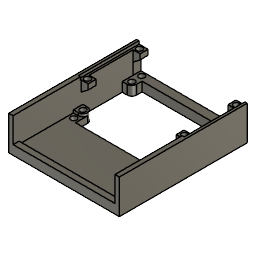
main (Autodesk Fusion 360 design; units mm, degrees)
Autodesk Fusion 360 part; units mm, degrees
note: some values were not read from the file. Set by a fixed rule: which sketch regions a step uses.
sketch "Szkic1" plane through (0, 0, 0) normal (0, 0, 1) x (1, 0, 0)
  line L0 (7.004, 84.481) -> (7.004, 88.113)
  arc A0 (3.502, 80.979) -> (7.004, 84.481) centre (3.502, 84.481) ccw
  line L1 (0, 80.979) -> (3.502, 80.979)
  line L2 (0, 0) -> (0, 88.113)
  line L3 (-0.2, 0) -> (-0.2, 88.113)
  line L4 (-3.5, 0) -> (-3.5, 88.113)
  line L5 (-3.5, 89.113) -> (-3.5, 95.113)
  line L6 (0, 95.113) -> (-3.5, 95.113)
  line L7 (-3.5, 89.113) -> (-3.5, 88.113)
  line L8 (0, 88.113) -> (76.073, 88.113)
  line L9 (-0.2, 88.113) -> (-0.2, 89.113)
  line L10 (0, 95.113) -> (76.073, 95.113)
  line L11 (76.273, 89.113) -> (76.273, 95.113)
  line L12 (76.073, 88.113) -> (76.073, 0)
  line L13 (76.273, 88.113) -> (76.273, 89.113)
  line L14 (76.273, 0) -> (76.273, 88.113)
  circle A1 centre (72.571, 84.481) radius 2.25
  arc A2 (69.069, 84.481) -> (72.571, 80.979) centre (72.571, 84.481) ccw
  line L15 (69.069, 84.481) -> (69.069, 88.113)
  line L16 (76.073, 80.979) -> (72.571, 80.979)
  circle A3 centre (3.502, 84.481) radius 2.25
  line L17 (0, -1) -> (-3.5, -1)
  line L18 (-3.5, -1) -> (-3.5, 0)
  line L19 (-0.2, 0) -> (-0.2, -1)
  line L20 (76.073, 0) -> (0, 0)
  line L21 (76.073, -1) -> (0, -1)
  arc A4 (3.502, 44.277) -> (3.502, 51.281) centre (3.502, 47.779) ccw
  line L22 (3.502, 51.281) -> (0, 51.281)
  line L23 (3.502, 44.277) -> (0, 44.277)
  circle A5 centre (3.502, 47.779) radius 2.25
  line L24 (72.571, 51.281) -> (76.073, 51.281)
  line L25 (72.571, 44.277) -> (76.073, 44.277)
  arc A6 (72.571, 51.281) -> (72.571, 44.277) centre (72.571, 47.779) ccw
  circle A7 centre (72.571, 47.779) radius 2.25
  line L26 (79.573, 88.113) -> (79.573, 0)
  line L27 (76.073, 95.113) -> (79.573, 95.113)
  line L28 (79.573, 95.113) -> (79.573, 89.113)
  line L29 (79.573, 89.113) -> (79.573, 88.113)
  line L30 (79.573, -1) -> (79.573, 0)
  line L31 (76.273, 0) -> (76.273, -1)
  line L32 (76.073, -1) -> (79.573, -1)
  line L33 (-0.2, 89.113) -> (-0.2, 95.113)
  line L34 (0, 88.113) -> (-0.2, 88.113)
  line L35 (76.073, 88.113) -> (76.273, 88.113)
  line L36 (76.073, 0) -> (76.273, 0)
  line L37 (0, 0) -> (-0.2, 0)
  line L38 (73.073, 0) -> (73.073, 3.5)
  line L39 (73.073, 3.5) -> (76.073, 3.5)
  line L40 (38.0365, 101.5763) -> (38.0365, -20) construction
  line L41 (3, 0) -> (3, 3.5)
  line L42 (3, 3.5) -> (0, 3.5)
  line L43 (69.069, 88.113) -> (69.069, 95.113)
  line L44 (7.004, 88.113) -> (7.004, 95.113)
  line L45 (82, 66.13) -> (-9, 66.13) construction
  circle A8 centre (3.502, 91.9192) radius 2.25
  circle A9 centre (3.502, 40.9192) radius 2.25
  circle A10 centre (72.571, 91.9192) radius 2.25
  circle A11 centre (72.571, 40.9192) radius 2.25
  line L46 (0, 3.5) -> (-0.2, 3.5)
  line L47 (76.073, 3.5) -> (76.273, 3.5)
  line L48 (0, 80.979) -> (-0.2, 80.979)
  line L49 (76.073, 80.979) -> (76.273, 80.979)
  line L50 (0, 44.277) -> (-0.2, 44.277)
  line L51 (0, 51.281) -> (-0.2, 51.281)
  line L52 (76.073, 51.281) -> (76.273, 51.281)
  line L53 (76.073, 44.277) -> (76.273, 44.277)
  line L54 (3, 3.5) -> (73.073, 3.5)
  dimension "d3" = 3
  dimension "d4" = 4.5
  dimension "d5" = 4.5
  dimension "d48" = 51
  constraint coincident L2.end L8.start
  constraint coincident L3.end L9.start
  constraint coincident L8.end L12.start
  constraint coincident L13.start L14.end
  constraint coincident L12.end L20.start
  constraint coincident L14.start L31.start
  constraint coincident L2.start L20.end
  constraint coincident L3.start L19.start
  constraint coincident L20 L38.start
  constraint perpendicular L20 L38
  constraint coincident L12 L39.end
  constraint perpendicular L12 L39
  constraint perpendicular L20 L40
  constraint symmetric L38.start L40 L41.start
  constraint symmetric L38.end L40 L41.end
  constraint symmetric L39.end L40 L42.end
  constraint coincident L15.end L43.start
  constraint coincident L10 L43.end
  constraint perpendicular L10 L43
  constraint coincident L0.end L44.start
  constraint coincident L10 L44.end
  constraint perpendicular L10 L44
  constraint perpendicular L4 L45
  constraint symmetric A3 A5 L45
  constraint symmetric L40 A8 A10
  constraint symmetric L40 A9 A11
  constraint coincident L3 L46.end
  constraint perpendicular L3 L46
  constraint coincident L14 L47.end
  constraint perpendicular L14 L47
  constraint coincident L1.start L48.start
  constraint coincident L3 L48.end
  constraint perpendicular L3 L48
  constraint coincident L16.start L49.start
  constraint perpendicular L14 L49
  constraint coincident L23.end L50.start
  constraint coincident L3 L50.end
  constraint perpendicular L3 L50
  constraint coincident L22.end L51.start
  constraint coincident L3 L51.end
  constraint perpendicular L3 L51
  constraint coincident L24.end L52.start
  constraint coincident L14 L52.end
  constraint perpendicular L14 L52
  constraint coincident L25.end L53.start
  constraint coincident L14 L53.end
  constraint perpendicular L14 L53
  measures "d3" distance of L38.end L39.end
  measures "d4" diameter of A8
  measures "d5" diameter of A9
  measures "d48" distance of A10.centre A11.centre
extrude "Wyciągnięcie proste2" add sketch "Szkic1" along normal blind 5
extrude "Wyciągnięcie proste3" add sketch "Szkic1" along normal blind 7 contours L0 A0 L1 L2 L8 | L8 L10 L43 L44 | L6 L8 L9 L10 L33 L34 L44 | L2 L3 L34 L48 | L8 L10 L11 L13 L27 L35 L43 | L8 L12 A2 L15 L16 | L3 L4 L5 L6 L7 L9 L17 L18 L19 L33 | L12 L14 L35 L49 | L2 A4 L22 L23 | L2 L3 L50 L51 | L11 L13 L14 L26 L27 L28 L29 L30 L31 L32 | L12 L14 L52 L53 | L12 L24 L25 A6 | L2 L20 L41 L42 | L2 L3 L37 L46 | L17 L19 L20 L21 L31 L32 L36 L37 | L12 L14 L36 L47 | L12 L20 L38 L39
extrude "Wyciągnięcie proste4" add sketch "Szkic1" along normal blind 25.8 contours L3 L4 L5 L6 L7 L9 L17 L18 L19 L33 | L11 L13 L14 L26 L27 L28 L29 L30 L31 L32
sketch "Szkic2" plane through (0, 95.113, 0) normal (0, 1, 0) x (-1, 0, 0)
  line L0 (-79.573, 0) -> (0, 0)
  line L1 (0, 0) -> (0, 7)
  line L2 (0, 7) -> (-76.273, 7)
  line L3 (-76.273, 7) -> (-76.273, 25.8)
  line L4 (-76.273, 25.8) -> (-79.573, 25.8)
  line L5 (-79.573, 25.8) -> (-79.573, 0)
sketch "Szkic3" plane through (0, 95.113, 0) normal (0, 1, 0) x (-1, 0, 0)
  line L0 (-79.573, 0) -> (0, 0)
  line L1 (0, 0) -> (0, 7)
  line L2 (0, 7) -> (-76.273, 7)
  line L3 (-76.273, 7) -> (-76.273, 25.8)
  line L4 (-76.273, 25.8) -> (-79.573, 25.8)
  line L5 (-79.573, 25.8) -> (-79.573, 0)
  line L6 (-38.0365, 31.6358) -> (-38.0365, -19.2) construction
  line L7 (-76.273, 23.6) -> (-69.069, 23.6)
  line L8 (-69.069, 23.6) -> (-69.069, 20.804)
  line L9 (-76.273, 13.6) -> (-76.273, 23.6)
  line L10 (-76.273, 25.8) -> (-79.573, 25.8)
  line L11 (-76.273, 13.6) -> (-69.069, 20.804)
  line L12 (-76.273, 13.6) -> (-66.085, 13.6) construction
  line L13 (0.2, 23.6) -> (-7.004, 23.6)
  line L14 (0.2, 13.6) -> (-7.004, 20.804)
  line L15 (-7.004, 23.6) -> (-7.004, 20.804)
  line L16 (0.2, 13.6) -> (0.2, 23.6)
  dimension "d12" = 10
  dimension "d13" = 2.2
  dimension "d14" = 45
  constraint perpendicular L0 L6
  constraint horizontal L7
  constraint vertical L8
  constraint vertical L9
  constraint coincident L3 L7.start
  constraint horizontal L12
  constraint symmetric L6 L7.start L13.start
  constraint symmetric L6 L7.end L13.end
  constraint symmetric L6 L9.start L14.start
  constraint symmetric L6 L8.end L14.end
  measures "d12" distance of L7.start L9.start
  measures "d13" distance of L7 L10
  measures "d14" angle of L11 L12
extrude "Wyciągnięcie proste5" add sketch "Szkic3" against normal blind 7 contours L3 L7 L8 L9 L11 | L13 L14 L15 L16
sketch "Szkic4" plane through (0, 0, 23.6) normal (0, 0, 1) x (-1, 0, 0)
  line L0 (-76.273, -95.113) -> (-69.069, -95.113)
  line L1 (-69.069, -95.113) -> (-69.069, -88.113)
  line L2 (-69.069, -88.113) -> (-76.273, -88.113)
  line L3 (-76.273, -88.113) -> (-76.273, -95.113)
  circle A0 centre (-74.5365, -92.113) radius 2.25
  line L4 (-76.273, -95.113) -> (-77.7365, -95.113)
  line L5 (-77.7365, -95.113) -> (-77.7365, -50.113)
  line L6 (-77.7365, -50.113) -> (-76.273, -50.113)
  line L7 (-76.273, -56.113) -> (-76.273, -50.113)
  circle A1 centre (-74.5365, -53.113) radius 2.25
  line L8 (-78.0365, -95.113) -> (-71.0365, -95.113)
  line L9 (-71.0365, -95.113) -> (-71.0365, -89.113)
  line L10 (-71.0365, -89.113) -> (-78.0365, -89.113)
  line L11 (-78.0365, -89.113) -> (-78.0365, -95.113)
  line L12 (-78.0365, -95.113) -> (-71.0365, -89.113) construction
  line L13 (-71.0365, -95.113) -> (-78.0365, -89.113) construction
  line L14 (-78.0365, -50.113) -> (-71.0365, -50.113)
  line L15 (-71.0365, -50.113) -> (-71.0365, -56.113)
  line L16 (-71.0365, -56.113) -> (-78.0365, -56.113)
  line L17 (-78.0365, -56.113) -> (-78.0365, -50.113)
  line L18 (-78.0365, -50.113) -> (-71.0365, -56.113) construction
  line L19 (-71.0365, -50.113) -> (-78.0365, -56.113) construction
  line L20 (-76.273, -95.113) -> (0, -95.113) construction
  line L21 (-38.0365, -105.87) -> (-38.0365, 20) construction
  line L22 (1.9635, -95.113) -> (-5.0365, -95.113)
  line L23 (-5.0365, -95.113) -> (-5.0365, -89.113)
  line L24 (-5.0365, -89.113) -> (1.9635, -89.113)
  circle A2 centre (-1.5365, -92.113) radius 2.25
  line L25 (1.6635, -95.113) -> (1.6635, -50.113)
  line L26 (-5.0365, -56.113) -> (1.9635, -56.113)
  line L27 (-5.0365, -50.113) -> (-5.0365, -56.113)
  line L28 (1.9635, -50.113) -> (-5.0365, -50.113)
  circle A3 centre (-1.5365, -53.113) radius 2.25
  line L29 (-76.273, -89.113) -> (-76.273, -56.113)
  line L30 (-76.273, -56.113) -> (-76.273, -89.113)
  line L31 (-76.273, -89.113) -> (-76.273, -95.113)
  line L32 (-77.7365, -95.113) -> (-77.7365, -50.113)
  line L33 (-76.273, -50.113) -> (-76.273, -56.113)
  line L34 (-76.273, -50.113) -> (-77.7365, -50.113)
  line L35 (-76.273, -95.113) -> (-76.273, -93.5438)
  line L36 (-76.273, -89.113) -> (-76.273, -90.6822)
  line L37 (-76.273, -95.113) -> (-71.0365, -95.113)
  line L38 (-76.273, -89.113) -> (-71.0365, -89.113)
  line L39 (-76.273, -56.113) -> (-71.0365, -56.113)
  line L40 (-71.0365, -56.113) -> (-76.273, -56.113)
  line L41 (-71.0365, -50.113) -> (-76.273, -50.113)
  line L42 (-76.273, -50.113) -> (-76.273, -51.6822)
  line L43 (-76.273, -56.113) -> (-76.273, -54.5438)
  line L44 (-5.0365, -56.113) -> (0.2, -56.113)
  line L45 (0.2, -56.113) -> (0.2, -89.113)
  line L46 (0.2, -56.113) -> (0.2, -54.5438)
  line L47 (-5.0365, -50.113) -> (-5.0365, -56.113)
  line L48 (-5.0365, -50.113) -> (0.2, -50.113)
  circle A4 centre (-1.5365, -53.113) radius 2.25
  line L49 (0.2, -50.113) -> (0.2, -51.6822)
  line L50 (1.6635, -50.113) -> (0.2, -50.113)
  line L51 (1.6635, -95.113) -> (1.6635, -50.113)
  line L52 (0.2, -95.113) -> (1.6635, -95.113)
  line L53 (0.2, -95.113) -> (-5.0365, -95.113)
  circle A5 centre (-1.5365, -92.113) radius 2.25
  line L54 (0.2, -95.113) -> (0.2, -93.5438)
  line L55 (0.2, -89.113) -> (0.2, -90.6822)
  line L56 (-5.0365, -95.113) -> (-5.0365, -89.113)
  line L57 (0.2, -89.113) -> (-5.0365, -89.113)
  line L58 (-71.0365, -50.113) -> (-77.7365, -50.113)
  line L59 (-77.7365, -50.113) -> (-77.7365, -49.613)
  line L60 (-77.7365, -49.613) -> (-71.0365, -49.613)
  line L61 (-71.0365, -49.613) -> (-71.0365, -50.113)
  line L62 (-5.0365, -49.613) -> (-5.0365, -50.113)
  line L63 (1.6635, -49.613) -> (-5.0365, -49.613)
  line L64 (1.6635, -50.113) -> (1.6635, -49.613)
  point P0 (-74.5365, -92.113)
  point P1 (-74.5365, -53.113)
  dimension "d17" = 4.5
  dimension "d19" = 3
  dimension "d20" = 45
  dimension "d21" = 3.2
  dimension "d23" = 4.5
  dimension "d24" = 39
  dimension "d29" = 7
  dimension "d30" = 7
  dimension "d31" = 6
  dimension "d32" = 36.5
  dimension "d37" = 0.5
  constraint horizontal L4
  constraint vertical L5
  constraint horizontal L6
  constraint coincident L0.start L3.end
  constraint vertical L7
  constraint horizontal L8
  constraint perpendicular L8 L9
  constraint parallel L8 L10
  constraint parallel L9 L11
  constraint coincident L12 P0
  constraint coincident L13 P0
  constraint coincident P0 A0.centre
  constraint horizontal L14
  constraint perpendicular L14 L15
  constraint parallel L14 L16
  constraint parallel L15 L17
  constraint coincident L18 P1
  constraint coincident L19 P1
  constraint coincident P1 A1.centre
  constraint perpendicular L20 L21
  constraint symmetric A0 L21 A2
  constraint symmetric L4.end L21 L25.start
  constraint symmetric L5.end L21 L25.end
  constraint symmetric A1 L21 A3
  constraint symmetric L8.start L21 L22.start
  constraint symmetric L8.end L21 L22.end
  constraint symmetric L9.end L21 L23.end
  constraint symmetric L10.end L21 L24.end
  constraint symmetric L14.start L21 L28.start
  constraint symmetric L14.end L21 L27.start
  constraint symmetric L15.end L21 L26.start
  constraint symmetric L16.end L21 L26.end
  constraint coincident L10 L29.start
  constraint coincident L3 L29.start
  constraint perpendicular L16 L29
  constraint coincident A0 L35.end
  constraint coincident L31 L35.end
  constraint coincident A0 L36.end
  constraint coincident L31 L36.end
  constraint perpendicular L9 L37
  constraint perpendicular L15 L39
  constraint perpendicular L7 L41
  constraint coincident A1 L42.end
  constraint coincident L7 L42.end
  constraint coincident A1 L43.end
  constraint coincident L7 L43.end
  constraint symmetric A0 L21 A5
  constraint symmetric L0.start L21 L52.start
  constraint symmetric L6.end L21 L48.end
  constraint symmetric L7.start L21 L44.end
  constraint symmetric A1 L21 A4
  constraint symmetric L21 L29.start L45.end
  constraint symmetric L21 L35.end L54.end
  constraint symmetric L21 L36.end L55.end
  constraint symmetric L21 L0.start L52.start
  constraint symmetric L21 L42.end L49.end
  constraint symmetric L21 L43.end L46.end
  constraint horizontal L58
  constraint vertical L59
  constraint horizontal L60
  constraint vertical L61
  constraint symmetric L21 L5.end L25.end
  constraint symmetric L21 L59.end L63.start
  constraint symmetric L21 L60.end L62.start
  measures "d17" diameter of A0
  measures "d19" distance of L0 P0
  measures "d20" distance of L0.start L6.end
  measures "d21" distance of P0 L5
  measures "d23" diameter of A1
  measures "d24" distance of P0 P1
  measures "d29" distance of L9.end L10.end
  measures "d30" distance of L15.end L16.end
  measures "d31" distance of L14.end L15.end
  measures "d32" distance of P0 L21
  measures "d37" distance of L14.end L60.end
extrude "Wyciągnięcie proste6" cut sketch "Szkic4" 1 faces at (4.6027, 90.7797, 23.6) against normal blind 10 contours L0 L3 A0 L8 L9 L10 L31 L35 L36 L37 L38 | L0 L1 L2 L3 L9 L10 L29 L30 L38 | L3 A0 L31 picked at (-73.0917, -91.9544)
extrude "Wyciągnięcie proste7" cut sketch "Szkic4" along normal blind 4 contours L3 A0 L4 L5 L8 L10 L31 L32 L35 L36 | L3 A0 L31 | L3 A0 L31 | L3 L5 L10 L16 L29 L30 L32 | L5 L6 L7 A1 L14 L16 L32 L33 L34 L42 L43 L58 | L6 L14 L34 L41 L58 L59 L60 L61 | L7 A1 L33 | L7 A1 L33 | L22 L24 A2 L25 L51 L52 A5 L54 L55 | L24 L25 L26 L45 L51 | A2 A5 | L25 L26 L28 A3 L46 A4 L49 L50 L51 | L28 L48 L50 L62 L63 L64 | A3 A4
extrude "Wyciągnięcie proste8" cut sketch "Szkic4" against normal blind 8 contours L3 A0 L31 | L3 A0 L31 | L7 A1 L33 | L7 A1 L33 | A2 A5 | A3 A4
extrude "Wyciągnięcie proste9" add sketch "Szkic4" against normal blind 8 contours L0 L3 A0 L8 L9 L10 L31 L35 L36 L37 L38 | L7 A1 L14 L15 L16 L33 L39 L40 L41 L42 L43 L58 | L22 L23 L24 A2 L53 A5 L54 L55 L56 L57 | L26 L27 L28 A3 L44 L46 L47 L48 A4 L49
sketch "Szkic5" plane through (0, 95.113, 0) normal (0, 1, 0) x (-1, 0, 0)
  line L0 (-77.7365, 23.6) -> (-77.7365, 25.8)
  line L1 (-77.7365, 25.8) -> (-79.573, 25.8)
  line L2 (-79.573, 25.8) -> (-79.573, 0)
  line L3 (-79.573, 0) -> (0, 0)
  line L4 (0, 0) -> (0, 7)
  line L5 (0, 7) -> (-76.273, 7)
  line L6 (-76.273, 7) -> (-76.273, 15.6)
  line L7 (-76.273, 15.6) -> (-71.0365, 15.6)
  line L8 (-71.0365, 15.6) -> (-71.0365, 23.6)
  line L9 (-71.0365, 23.6) -> (-77.7365, 23.6)
  line L10 (-76.273, 15.6) -> (-71.0365, 19.6)
  line L11 (-69.069, 5) -> (-7.004, 5) construction
  line L12 (-38.0365, 29.2995) -> (-38.0365, -9) construction
  line L13 (0.2, 15.6) -> (-5.0365, 19.6)
  line L14 (-5.0365, 23.6) -> (-5.0365, 15.6) construction
  line L15 (-5.0365, 19.6) -> (-5.0365, 15.6)
  line L16 (-5.0365, 15.6) -> (0.2, 15.6)
  point P0 (-5.0365, 15.6)
  constraint coincident L6.end L7.start
  constraint midpoint L8 L10.end
  constraint perpendicular L11 L12
  constraint symmetric L6.end L12 L13.start
  constraint symmetric L10.end L12 L13.end
  constraint coincident P0 L14.end
  constraint parallel L14 L15
extrude "Wyciągnięcie proste10" cut sketch "Szkic5" against normal blind 52 contours L7 L8 L10 | L13 L15 L16
sketch "Szkic6" plane through (0, 0, 0) normal (0, 0, -1) x (1, 0, 0)
  circle A0 centre (72.571, -47.779) radius 2.25
  circle A1 centre (3.502, -84.481) radius 2.25
  circle A2 centre (72.571, -91.9192) radius 2.25
  circle A3 centre (3.502, -91.9192) radius 2.25
  circle A4 centre (3.502, -47.779) radius 2.25
  circle A5 centre (72.571, -84.481) radius 2.25
  circle A6 centre (3.502, -40.9192) radius 2.25
  circle A7 centre (72.571, -40.9192) radius 2.25
  line L0 (79.573, 1) -> (-3.5, 1)
  line L1 (-3.5, 1) -> (-3.5, 0)
  line L2 (-3.5, 0) -> (-3.5, -88.113)
  line L3 (-3.5, -88.113) -> (-3.5, -89.113)
  line L4 (-3.5, -89.113) -> (-3.5, -95.113)
  line L5 (-3.5, -95.113) -> (0, -95.113)
  line L6 (0, -95.113) -> (79.573, -95.113)
  line L7 (79.573, -95.113) -> (79.573, 1)
  circle A8 centre (72.571, -91.9192) radius 3.502
  line L8 (69.069, -88.113) -> (69.069, -95.113)
  line L9 (38.0365, -94.1692) -> (72.571, -94.1692)
  arc A9 (72.571, -44.277) -> (72.571, -51.281) centre (72.571, -47.779) ccw
  line L10 (69.069, -47.779) -> (69.069, -40.9192)
  line L11 (38.0365, -38.6692) -> (72.571, -38.6692)
  line L12 (69.069, -40.9192) -> (69.069, -38.6692)
  line L13 (38.0365, -101.5763) -> (38.0365, 20) construction
  line L14 (38.0365, -94.1692) -> (3.502, -94.1692)
  line L15 (7.004, -47.779) -> (7.004, -40.9192)
  line L16 (7.004, -40.9192) -> (7.004, -38.6692)
  line L17 (38.0365, -38.6692) -> (3.502, -38.6692)
  line L18 (7.004, -94.1692) -> (69.069, -94.1692)
  line L19 (69.069, -94.1692) -> (69.069, -88.113)
  line L20 (7.004, -88.113) -> (7.004, -94.1692)
  line L21 (72.571, -51.281) -> (76.073, -51.281)
  line L22 (76.073, -51.281) -> (76.073, -80.979)
  arc A10 (72.571, -80.979) -> (69.069, -84.481) centre (72.571, -84.481) ccw
  line L23 (76.073, -80.979) -> (72.571, -80.979)
  line L24 (69.069, -88.113) -> (69.069, -84.481)
  arc A11 (72.571, -80.979) -> (69.069, -84.481) centre (72.571, -84.481) ccw
  arc A12 (71.864, -44.3491) -> (73.278, -44.3491) centre (72.571, -40.9192) ccw
  line L25 (69.069, -40.9192) -> (69.069, -38.6692)
  arc A13 (69.069, -47.779) -> (72.571, -51.281) centre (72.571, -47.779) ccw
  arc A14 (73.278, -44.3491) -> (71.864, -44.3491) centre (72.571, -47.779) ccw
  line L26 (38.0365, -101.5763) -> (38.0365, 20)
  line L27 (0, -51.281) -> (0, -80.979)
  line L28 (3.502, -51.281) -> (0, -51.281)
  arc A15 (3.502, -51.281) -> (7.004, -47.779) centre (3.502, -47.779) ccw
  line L29 (7.004, -47.779) -> (7.004, -40.9192)
  line L30 (7.004, -40.9192) -> (7.004, -38.6692)
  line L31 (0, -80.979) -> (3.502, -80.979)
  arc A16 (7.004, -84.481) -> (3.502, -80.979) centre (3.502, -84.481) ccw
  line L32 (7.004, -88.113) -> (7.004, -84.481)
  line L33 (7.004, -88.6692) -> (38.0365, -88.6692)
  line L34 (69.069, -88.6692) -> (38.0365, -88.6692)
  point P0 (38.0365, -101.5763)
  point P1 (76.073, -51.281)
  point P2 (76.073, -80.979)
  dimension "d50" = 50
  constraint concentric A2 A8
  constraint tangent A8 L8
  constraint coincident A2 L9.end
  constraint tangent A2 L9
  constraint concentric A7 A12
  constraint midpoint A9 L10.start
  constraint tangent L10 A12
  constraint vertical L10
  constraint coincident A7 L11.end
  constraint tangent A7 L11
  constraint coincident L11 L12.end
  constraint tangent L12 A12
  constraint coincident P0 L13.start
  constraint perpendicular L0 L13
  constraint coincident L9.start L13
  constraint perpendicular L9 L13
  constraint coincident L11.start L13
  constraint perpendicular L11 L13
  constraint symmetric L9.start L13 L14.start
  constraint symmetric L9.end L13 L14.end
  constraint symmetric L10.start L13 L15.start
  constraint symmetric L10.end L13 L15.end
  constraint symmetric L11.start L13 L17.start
  constraint symmetric L11.end L13 L17.end
  constraint symmetric L12.end L13 L16.end
  constraint horizontal L18
  constraint vertical L19
  constraint vertical L20
  constraint coincident L8.start L19.end
  constraint coincident L14 L18.start
  constraint concentric A9 A13
  constraint coincident A9.end L21.start
  constraint coincident P1 L21.end
  constraint coincident P2 L22.end
  constraint coincident A10.start L23.end
  constraint concentric A10 A11
  constraint coincident A10.end L24.end
  constraint perpendicular L11 L25
  constraint concentric A13 A14
  constraint symmetric A9.end L26 L28.start
  constraint symmetric L10.start L26 L15.start
  constraint symmetric L10.end L26 L15.end
  constraint symmetric L12.end L26 L16.end
  constraint symmetric L8.start L26 L20.start
  constraint symmetric P1 L26 L27.start
  constraint symmetric P2 L26 L27.end
  constraint symmetric A10.start L26 L31.end
  constraint symmetric A10.end L26 A16.start
  constraint symmetric A11 L26 A16
  constraint symmetric A13 L26 A15
  constraint coincident L20 L33.start
  constraint coincident L26 L33.end
  constraint perpendicular L26 L33
  constraint symmetric L13 L33.start L34.start
  constraint symmetric L13 L33.end L34.end
  measures "d50" distance of L17 L33
extrude "Wyciągnięcie proste11" cut sketch "Szkic6" against normal blind 8 contours L15 L16 L17 L20 L26 L27 L28 A15 L29 L30 L31 A16 L32 L33 | L8 A9 L10 L11 L12 L19 L21 L22 A10 L23 L24 A11 L25 A13 L26 L34
extrude "Wyciągnięcie proste12" cut 2 faces at (76.2063, 61.1803, 5) (-0.1333, 71.0797, 5) along direction (0, 0, -1) blind 7
extrude "Wyciągnięcie proste13" add sketch "Szkic1" along normal blind 7 contours L20 L38 L41 L54
move_body "Przesuń1" bodies 1 to x (1, 0, 0) y (0, 1, 0) z (0, 0, 1) at (-38.0365, -38.6692, 0)
move_body "Przesuń2" bodies 1 to x (1, 0, 0) y (0, 1, 0) z (0, 0, 1) at (0, 20, 0)
